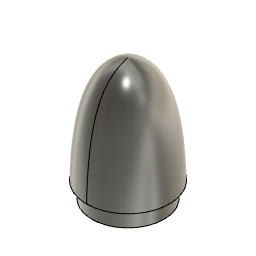
nozzle v2 v4 (Autodesk Fusion 360 design; units mm, degrees)
Autodesk Fusion 360 part; units mm, degrees
sketch "Sketch1" plane through (0, 0, 0) normal (1, 0, 0) x (0, 1, 0)
  line L0 (0, 0) -> (-39, 0) construction
  line L1 (0, 0) -> (0, 100) construction
  spline S0 degree 5 poles (-39, 0) (-38.942, 3.3768) (-38.7689, 10.0218) (-38.3385, 19.6635) (-37.4173, 31.8566) (-35.642, 45.9083) (-33.1709, 58.6335) (-29.9149, 69.8616) (-25.7862, 79.4253) (-20.7237, 87.2084) (-14.7404, 93.2356) (-9.2559, 96.7263) (-4.7703, 98.6346) (-1.6172, 99.5966) (0, 100) knots 0 0 0 0 0 0 0.1 0.2 0.3 0.4 0.5 0.6 0.7 0.8 0.9 1 1 1 1 1 1
  spline S1 degree 5 poles (-30, 0) (-30.0249, 3.0944) (-30.0256, 9.1895) (-29.8796, 18.0509) (-29.3857, 29.2944) (-28.2311, 42.3217) (-26.4766, 54.2023) (-24.0438, 64.7865) (-20.8549, 73.9254) (-16.8534, 81.5112) (-12.0463, 87.557) (-7.5889, 91.2244) (-3.9193, 93.3509) (-1.3302, 94.4957) (0, 95) knots 0 0 0 0 0 0 0.1 0.2 0.3 0.4 0.5 0.6 0.7 0.8 0.9 1 1 1 1 1 1
  line L2 (0, 95) -> (0, 100)
  line L3 (-30, 0) -> (-39, 0)
  point P0 (-25, 80)
  point P1 (-20, 75)
  dimension "d5" = 39
  dimension "d6" = 100
  constraint coincident L0.start L1.start
  constraint horizontal L0
  constraint perpendicular L0 L1
  constraint coincident L0 S1.start
  constraint coincident L1 S1.end
  measures "d5" distance of L0.start L0.end
  measures "d6" distance of L0.start L1.end
revolve "Revolve1" add sketch "Sketch1" angle 360 about axis through (0, 0, 0) along (0, 0, 1)
sketch "Sketch2" plane through (0, 0, 0) normal (0, 0, 1) x (1, 0, 0)
  circle A0 centre (0, 0) radius 34
  circle A1 centre (0, 0) radius 30
  dimension "d8" = 68
  dimension "d9" = 60
  constraint coincident A0.centre A1.centre
  measures "d8" diameter of A0
  measures "d9" diameter of A1
extrude "Extrude1" add sketch "Sketch2" against normal blind 15
sketch "Sketch3" plane through (0, 0, 0) normal (0, 0, 1) x (1, 0, 0)
  line L0 (-30, -5) -> (30, -5)
  line L1 (30, -5) -> (30, 5)
  line L2 (30, 5) -> (-30, 5)
  line L3 (-30, 5) -> (-30, -5)
  constraint horizontal L0
  constraint vertical L1
  constraint horizontal L2
  constraint vertical L3
extrude "Extrude2" add sketch "Sketch3" against normal blind 15
equation "innerdi = 68 mm"
equation "noseconeheight = 100 mm"
equation "d6 = noseconeheight"
equation "d8 = innerdi"
equation "d9 = innerdi - 8 mm"
